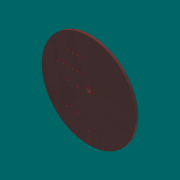
# Autodesk Inventor part: 知能ロボコンターンテーブル1.1
Saved by Autodesk Inventor 2013 (Build 170138000, 138)
## iProperties
Created: 2014-05-11
Part Number: 知能ロボコンターンテーブル1.1
Material: アセタール樹脂、白
Document SubType Name: Modeling
Designer: horumo136
Density: 1 g/cm^3
Author: horumo136
Autodesk Inventor part; units mm, degrees
ref_plane "YZ Plane" through (0, 0, 0) normal (1, 0, 0) x (0, 1, 0)
ref_plane "XZ Plane" through (0, 0, 0) normal (0, 1, 0) x (-1, 0, 0)
ref_plane "XY Plane" through (0, 0, 0) normal (0, 0, 1) x (1, 0, 0)
sketch "スケッチ1" plane through (0, 0, 0) normal (0, 1, 0) x (-1, 0, 0)
  circle A0 centre (0, 0) radius 100
  dimension "d0" = 200
  constraints: 1 centre point, 1 coincident
  measures "d0" diameter of A0
extrude "押し出し1" add sketch "スケッチ1" along normal blind 5
sketch "スケッチ12" plane through (0, 5, 0) normal (0, 1, 0) x (1, 0, 0)
  circle A0 centre (0, 0) radius 100 projected
  circle A1 centre (0, 0) radius 4
  circle A2 centre (0, 0) radius 5
  circle A3 centre (0, 0) radius 6
  circle A4 centre (0, 6) radius 1
  circle A5 centre (-4.2426, 4.2426) radius 1
  circle A6 centre (-6, 0) radius 1
  circle A7 centre (-4.2426, -4.2426) radius 1
  circle A8 centre (0, -6) radius 1
  circle A9 centre (4.2426, -4.2426) radius 1
  circle A10 centre (6, 0) radius 1
  circle A11 centre (4.2426, 4.2426) radius 1
  dimension "d94" = 12
  dimension "d92" = 8
  dimension "d93" = 10
  dimension "d95" = 2
  dimension "d98" = 360
  constraints: 10 centre point, 3 coincident, 1 vertical alignment, 19 other
  measures "d92" diameter of A1
  measures "d93" diameter of A2
  measures "d95" diameter of A4
hole "穴5" at (-6, 5, 0) at (-4.2426, 5, 4.2426) at (0, 5, 6) at (0, 5, -6) at (4.2426, 5, -4.2426) at (6, 5, 0) at (4.2426, 5, 4.2426) at (-4.2426, 5, -4.2426) direction (0, -1, 0) diameter 2.1 depth 8 tip angle 118
sketch "スケッチ13" plane through (0, 5, 0) normal (0, 1, 0) x (1, 0, 0)
  circle A0 centre (0, 0) radius 100 projected
  circle A1 centre (0, 0) radius 4
  dimension "d107" = 8
  constraints: 1 centre point, 1 coincident
  measures "d107" diameter of A1
extrude "押し出し4" cut sketch "スケッチ13" against normal blind 8 contours A1
sketch "スケッチ14" plane through (0, 5, 0) normal (0, 1, 0) x (1, 0, 0)
  circle A0 centre (0, 0) radius 100 projected
  line L0 (0, 0) -> (0, 63)
  line L1 (0, 63) -> (0, 73)
  line L2 (0, 73) -> (0, 93)
  line L3 (0, 73) -> (30, 73)
  line L4 (0, 73) -> (-30, 73)
  line L5 (-30, 73) -> (30, 73)
  line L6 (30, 73) -> (30, 93)
  line L7 (30, 93) -> (-30, 93)
  line L8 (-30, 93) -> (-30, 73)
  line L9 (0, 0) -> (0, -38.43)
  line L10 (0, -38.43) -> (-14.5, -38.43)
  line L11 (-14.5, -38.43) -> (-14.5, -23.43)
  line L12 (-14.5, -23.43) -> (-24.5, -23.43)
  line L13 (-24.5, -23.43) -> (-34.5, -23.43)
  line L14 (-34.5, -23.43) -> (-44.5, -23.43)
  line L15 (-44.5, -23.43) -> (-54.5, -23.43)
  line L16 (-54.5, -23.43) -> (-64.5, -23.43)
  line L17 (-24.5, -53.43) -> (-34.5, -53.43)
  line L18 (-34.5, -53.43) -> (-44.5, -53.43)
  line L19 (-44.5, -53.43) -> (-54.5, -53.43)
  line L20 (-54.5, -53.43) -> (-64.5, -53.43)
  point P0 (-14.5, -53.43)
  point P1 (-7.25, -38.43)
  dimension "d110" = 63
  dimension "d111" = 10
  dimension "d112" = 20
  dimension "d114" = 30
  dimension "d115" = 30
  dimension "d117" = 14.5
  dimension "d118" = 15
  dimension "d119" = 10
  dimension "d120" = 10
  dimension "d121" = 10
  dimension "d122" = 10
  dimension "d123" = 10
  dimension "d143" = 111.43
  constraints: 42 end point, 21 coincident, 11 symmetric about line, 8 parallel, 4 perpendicular, 3 collinear, 1 horizontal, 1 midpoint, 1 vertical
  measures "d110" distance of L0.start L0.end
  measures "d111" distance of L0.end L1.end
  measures "d112" distance of L1.end L2.end
  measures "d114" distance of L1.end L3.end
  measures "d115" distance of L1.end L4.end
  measures "d117" distance of L9.end L10.end
  measures "d118" distance of L10.end L11.end
  measures "d119" distance of L11.end L12.end
  measures "d120" distance of L12.end L13.end
  measures "d121" distance of L13.end L14.end
  measures "d122" distance of L14.end L15.end
  measures "d123" distance of L15.end L16.end
  measures "d143" distance between parallel lines of L10 L4
hole "穴6" at (-30, 5, -93) at (-30, 5, -73) at (0, 5, -93) at (0, 5, -73) at (30, 5, -73) at (30, 5, -93) at (-64.5, 5, 23.43) at (-54.5, 5, 23.43) at (-44.5, 5, 23.43) at (-34.5, 5, 23.43) at (-24.5, 5, 23.43) at (-14.5, 5, 23.43) at (-64.5, 5, 53.43) at (-54.5, 5, 53.43) at (-44.5, 5, 53.43) at (-34.5, 5, 53.43) at (-24.5, 5, 53.43) at (-14.5, 5, 53.43) at (-30, 5, -93) at (-30, 5, -73) direction (0, -1, 0) diameter 3 depth 8 tip angle 118
sketch "スケッチ16" plane through (0, 5, 0) normal (0, 1, 0) x (1, 0, 0)
  circle A0 centre (-64.5, -53.43) radius 1.5 projected
  circle A1 centre (30, 73) radius 1.5 projected
  circle A2 centre (-30, 73) radius 1.5 projected
  circle A3 centre (-54.5, -53.43) radius 1.5 projected
  circle A4 centre (0, 0) radius 100 projected
  circle A5 centre (0, 0) radius 78
  circle A6 centre (0, 0) radius 90
  circle A7 centre (-54.5, -53.43) radius 1.5
  circle A8 centre (-64.5, -53.43) radius 1.5
  circle A9 centre (-30, 73) radius 1.5
  circle A10 centre (30, 73) radius 1.5
  dimension "d145" = 156
  dimension "d147" = 180
  constraints: 6 centre point, 6 coincident, 2 concentric
  measures "d145" diameter of A5
  measures "d147" diameter of A6
extrude "押し出し7" add sketch "スケッチ16" against normal blind 5 contours A0 | A1 A5 | A5 A1 | A5 A2 | A2 A5 | A3
sketch "スケッチ17" plane through (0, 0, 0) normal (0, -1, 0) x (1, 0, 0)
  line L0 (-50.2739, -0.7823) -> (-20.2739, -0.7823)
  line L1 (-20.2739, -0.7823) -> (-20.2739, -54.7823)
  line L2 (-20.2739, -54.7823) -> (-50.2739, -54.7823)
  line L3 (-50.2739, -54.7823) -> (-50.2739, -0.7823)
  point P0 (-47.2739, -3.7823)
  point P1 (-47.2739, -51.7823)
  point P2 (-23.2739, -51.7823)
  point P3 (-23.2739, -3.7823)
  dimension "d150" = 30
  dimension "d151" = 54
  dimension "d153" = 3
  dimension "d154" = 48
  dimension "d155" = 3
  dimension "d156" = 3
  dimension "d157" = 24
  dimension "d158" = 24
  dimension "d159" = 3
  dimension "d160" = 48
  constraints: 8 end point, 2 parallel, 1 horizontal, 1 perpendicular
  measures "d150" distance of L1.end L2.end
  measures "d151" distance of L0.end L1.end
  measures "d153" distance from line of point (-23.274, -3.782) L1
  measures "d154" distance of point (-23.274, -51.782) point (-23.274, -3.782)
  measures "d155" distance from line of L0 point (-47.274, -3.782)
  measures "d156" distance from line of L0 point (-23.274, -3.782)
  measures "d157" distance of point (-47.274, -51.782) point (-23.274, -51.782)
  measures "d158" distance of point (-23.274, -3.782) point (-47.274, -3.782)
  measures "d159" distance from line of L1 point (-23.274, -51.782)
  measures "d160" distance of point (-47.274, -51.782) point (-47.274, -3.782)
hole "穴7" at (-47.2739, 0, -3.7823) at (-47.2739, 0, -51.7823) at (-23.2739, 0, -51.7823) at (-23.2739, 0, -3.7823) direction (0, 1, 0) diameter 3.2 depth 8 tip angle 118
